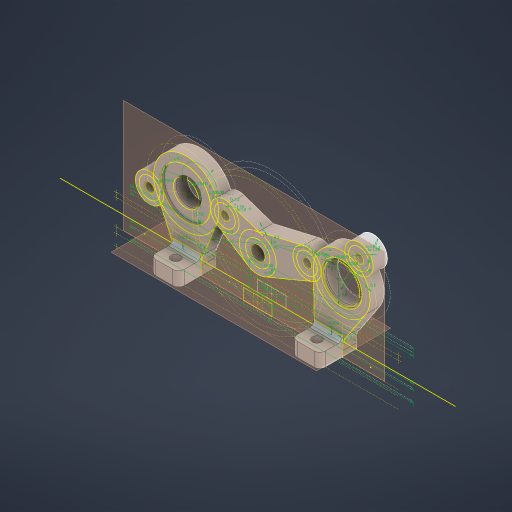
# Autodesk Inventor part: Motormount
Saved by Autodesk Inventor 2023.5 (Build 275446000, 446)
## iProperties
Created: 2024-12-07
Part Number: Motormount
Material: 一般
Document SubType Name: Modeling
Designer: IshiiLabHonda
Density: 1 g/cm^3
Appearance: 既定
Author: IshiiLabHonda
Autodesk Inventor part; units mm, degrees
ref_plane "YZ Plane" through (0, 0, 0) normal (1, 0, 0) x (0, 1, 0)
ref_plane "XZ Plane" through (0, 0, 0) normal (0, 1, 0) x (-1, 0, 0)
ref_plane "XY Plane" through (0, 0, 0) normal (0, 0, 1) x (1, 0, 0)
sketch "blueprint" plane through (0, 0, 0) normal (0, 0, 1) x (1, 0, 0)
  line L0 (0, 0) -> (0, 1) construction
  line L1 (0, 0) -> (1, 0) construction
  circle A0 centre (0, 0) radius 1.25
  circle A1 centre (0, 0) radius 11.5 construction
  line L2 (-25, -11.5) -> (25, -11.5) construction
  line L3 (-25, -9.5) -> (25, -9.5) construction
  line L4 (-25, -8.5) -> (25, -8.5) construction
  line L5 (-25, -4) -> (25, -4) construction
  circle A2 centre (0, 0) radius 10.65 construction
  circle A3 centre (-12.6949, 2.8) radius 2.25
  circle A4 centre (14.8381, 2.8) radius 4.35 construction
  circle A5 centre (14.8381, 2.8) radius 3.5 construction
  line L6 (-25, -3.2) -> (25, -3.2) construction
  circle A6 centre (-12.6949, 2.8) radius 4.25 construction
  circle A7 centre (-19.1553, 0.4486) radius 0.625 construction
  circle A8 centre (-5.8199, 2.8) radius 0.625 construction
  circle A9 centre (-12.6949, 2.8) radius 6.875 construction
  circle A10 centre (-19.1553, 0.4486) radius 1.825
  circle A11 centre (-5.8199, 2.8) radius 1.825
  circle A12 centre (14.8381, 2.8) radius 5
  circle A13 centre (14.8381, 2.8) radius 6.125 construction
  circle A14 centre (17.9006, 8.1044) radius 0.625 construction
  circle A15 centre (8.7131, 2.8) radius 0.625 construction
  circle A16 centre (17.9006, 8.1044) radius 1.825
  circle A17 centre (-19.1553, 0.4486) radius 0.8
  circle A18 centre (-5.8199, 2.8) radius 0.8
  circle A19 centre (17.9006, 8.1044) radius 0.8
  circle A20 centre (-19.1553, 0.4486) radius 2.5
  circle A21 centre (-5.8199, 2.8) radius 2.5
  circle A22 centre (17.9006, 8.1044) radius 2.5
  circle A23 centre (14.8381, 2.8) radius 3.6
  circle A24 centre (0, 0) radius 3.25
  line L7 (-15, -4) -> (-15, -8.5) construction
  line L8 (15, -4) -> (15, -8.5) construction
  line L9 (-10, -8.5) -> (-10, -6)
  line L10 (-15, -8.5) -> (-15, -6)
  line L11 (-15, -6) -> (-10, -6)
  line L12 (-12.5, -6) -> (-12.5, -8.5)
  line L13 (-13.3, -6) -> (-13.3, -8.5)
  line L14 (-11.7, -6) -> (-11.7, -8.5)
  line L15 (10, -8.5) -> (10, -6)
  line L16 (15, -8.5) -> (15, -6)
  line L17 (15, -6) -> (10, -6)
  line L18 (12.5, -6) -> (12.5, -8.5)
  line L19 (13.3, -6) -> (13.3, -8.5)
  line L20 (11.7, -6) -> (11.7, -8.5)
  line L21 (-15, -8.5) -> (-10, -8.5)
  line L22 (10, -8.5) -> (15, -8.5)
  circle A25 centre (8.7131, 2.8) radius 1.825
  line L23 (-12.6949, 2.8) -> (-19.1553, 0.4486) construction
  line L24 (-12.6949, 2.8) -> (-5.8199, 2.8) construction
  line L25 (14.8381, 2.8) -> (8.7131, 2.8) construction
  circle A26 centre (-12.6949, 2.8) radius 5.75
  line L26 (-2.5, -6.5) -> (2.5, -6.5)
  line L27 (2.5, -6.5) -> (2.5, -8.5)
  line L28 (2.5, -8.5) -> (-2.5, -8.5)
  line L29 (-2.5, -8.5) -> (-2.5, -6.5)
  line L30 (-2.5, -6.5) -> (2.5, -8.5) construction
  line L31 (2.5, -6.5) -> (-2.5, -8.5) construction
  line L32 (0, -6.5) -> (0, -8.5) construction
  line L33 (-0.8, -6.5) -> (-0.8, -8.5) construction
  line L34 (0.8, -6.5) -> (0.8, -8.5) construction
  circle A27 centre (8.7131, 2.8) radius 0.8
  circle A28 centre (8.7131, 2.8) radius 2.5
  line L35 (17.9006, 8.1044) -> (14.8381, 2.8) construction
  circle A29 centre (0, 0) radius 2.15
  circle A30 centre (14.8381, 2.8) radius 3 construction
  circle A31 centre (14.8381, 2.8) radius 3.2
  circle A32 centre (-12.6949, 2.8) radius 4.35
  point P0 (18.8457, 5.7899)
  point P1 (15.4237, 7.7656)
  point P2 (0, -8.5)
  point P3 (-6.4807, -9.5)
  point P4 (6.4807, -9.5)
  point P5 (0, -7.5)
  point P6 (-17.0702, -0.9308)
  point P7 (-7.3074, 0.7907)
  point P8 (-7.3074, 4.8093)
  point P9 (-18.4447, 2.8455)
  point P10 (11.284, 2.5721)
  point P11 (11.284, 2.0279)
  point P12 (16.9793, 5.3162)
  point P13 (16.5081, 5.5882)
  dimension "d0" = 1
  dimension "d1" = 1
  dimension "d2" = 2.5
  dimension "d3" = 23
  dimension "d4" = 50
  dimension "d5" = 50
  dimension "d6" = 2
  dimension "d7" = 50
  dimension "d9" = 1
  dimension "d10" = 50
  dimension "d12" = 4.5
  dimension "d13" = 21.3
  dimension "d14" = 4.5
  dimension "d15" = 8.7
  dimension "d17" = 0.1
  dimension "d18" = 0.1
  dimension "d20" = 7
  dimension "d21" = 50
  dimension "d22" = 0.8
  dimension "d23" = 8.5
  dimension "d26" = 1.25
  dimension "d27" = 1.25
  dimension "d28" = 1.2
  dimension "d29" = 1.2
  dimension "d31" = 1.5
  dimension "d32" = 1.25
  dimension "d33" = 1.25
  dimension "d34" = 1.2
  dimension "d37" = 0.5
  dimension "d40" = 1.6
  dimension "d41" = 1.6
  dimension "d43" = 1.6
  dimension "d49" = 2
  dimension "d56" = 30
  dimension "d90" = 2.5
  dimension "d92" = 5
  dimension "d93" = 1.6
  dimension "d104" = 1.2
  dimension "d105" = 5
  dimension "d106" = 1.6
  dimension "d107" = 2.5
  dimension "d129" = 5
  dimension "d130" = 5
  dimension "d132" = 5
  dimension "d155" = 25
  dimension "d158" = 1.5
  dimension "d160" = 0.5
  dimension "d161" = 200
  dimension "d166" = 1.6
  dimension "d167" = 5
  dimension "d168" = 2
  dimension "d178" = 1.6
  dimension "d179" = 5
  dimension "d181" = 6
  dimension "d187" = 1.75
  dimension "d196" = 4.3
  dimension "d218" = 10.6088
  dimension "d219" = 13.5411
  dimension "d220" = 120
  dimension "d221" = 6
  dimension "d237" = 0.1
  dimension "d238" = 6
  dimension "d239" = 0.2
  dimension "d247" = 0.1
  constraints: 70 end point, 33 centre point, 28 coincident, 16 point on line, 10 parallel, 8 midpoint, 7 vertical, 6 point on circle, 5 symmetric about line, 4 perpendicular, 3 horizontal, 1 tangent, 18 other
  measures "d0" distance of L0.start L0.end
  measures "d1" distance of L0.start L1.end
  measures "d2" diameter of A0
  measures "d3" diameter of A1
  measures "d4" distance of L2.start L2.end
  measures "d5" distance of L3.start L3.end
  measures "d6" distance between parallel lines of L2 L3
  measures "d7" distance of point (-25, -8.5) point (25, -8.5)
  measures "d10" distance of L5.start L5.end
  measures "d13" diameter of A2
  measures "d14" diameter of A3
  measures "d15" diameter of A4
  measures "d20" diameter of A5
  measures "d21" distance of L6.start L6.end
  measures "d22" distance between parallel lines of L5 L6
  measures "d23" diameter of A6
  measures "d26" diameter of A8
  measures "d27" diameter of A7
  measures "d28" radial gap between concentric circles of A10 A7
  measures "d29" radial gap between concentric circles of A11 A8
  measures "d31" radial gap between concentric circles of A12 A5
  measures "d32" diameter of A14
  measures "d33" diameter of A15
  measures "d34" radial gap between concentric circles of A14 A16
  measures "d40" diameter of A17
  measures "d41" diameter of A18
  measures "d43" diameter of A19
  measures "d49" radial gap between concentric circles of A24 A0
  measures "d56" distance between parallel lines of L8 L7
  measures "d90" distance of L10.start L10.end
  measures "d92" distance between parallel lines of L9 L10
  measures "d93" distance between parallel lines of L14 L13
  measures "d104" radial gap between concentric circles of A25 A15
  measures "d105" distance between parallel lines of L16 L15
  measures "d106" distance between parallel lines of L19 L20
  measures "d107" distance of L15.start L15.end
  measures "d129" diameter of A20
  measures "d130" diameter of A21
  measures "d132" diameter of A22
  measures "d155" distance between parallel lines of L18 L12
  measures "d158" radial gap between concentric circles of A26 A6
  measures "d166" distance between parallel lines of L33 L34
  measures "d167" distance between parallel lines of L27 L29
  measures "d168" distance between parallel lines of L26 L28
  measures "d178" diameter of A27
  measures "d179" diameter of A28
  measures "d181" distance between parallel lines of L6 L25
  measures "d187" distance edge to line of A6 L6
  measures "d196" diameter of A29
  measures "d218" distance of A14.centre L25.end
  measures "d219" distance of A7.centre A18.centre
  measures "d220" angle of L25 L35
  measures "d221" distance from line of A3.centre L6
  measures "d237" radial gap between concentric circles of A5 A23
  measures "d238" diameter of A30
  measures "d239" radial gap between concentric circles of A30 A31
  measures "d247" radial gap between concentric circles of A6 A32
sketch "スケッチ5" plane through (0, 0, 0) normal (0, 0, 1) x (1, 0, 0)
  circle A0 centre (0, 0) radius 10.65 construction
  circle A1 centre (0, 0) radius 11.5 construction
  line L0 (-25, -3.2) -> (25, -3.2) construction
  line L1 (-25, -4) -> (25, -4) construction
  line L2 (-25, -8.5) -> (25, -8.5) construction
  line L3 (-25, -9.5) -> (25, -9.5) construction
  line L4 (-25, -11.5) -> (25, -11.5) construction
  line L5 (0, 0) -> (1, 0) construction
  circle A2 centre (0, 0) radius 1.25 projected
  line L6 (0, 0) -> (0, 1) construction
  circle A3 centre (-5.8199, 2.8) radius 0.625 construction
  circle A4 centre (-5.8199, 2.8) radius 0.8 projected
  circle A5 centre (-5.8199, 2.8) radius 1.825 construction
  circle A6 centre (-5.8199, 2.8) radius 2.5 projected
  line L7 (-12.6949, 2.8) -> (-5.8199, 2.8) construction
  circle A7 centre (-12.6949, 2.8) radius 2.25 projected
  circle A8 centre (-12.6949, 2.8) radius 4.25 construction
  circle A9 centre (-12.6949, 2.8) radius 5.75 projected
  circle A10 centre (-12.6949, 2.8) radius 6.875 construction
  line L8 (-12.6949, 2.8) -> (-19.1553, 0.4486) construction
  circle A11 centre (-19.1553, 0.4486) radius 2.5 projected
  circle A12 centre (14.8381, 2.8) radius 3.5 construction
  circle A13 centre (14.8381, 2.8) radius 4.35 construction
  circle A14 centre (-19.1553, 0.4486) radius 0.625 construction
  circle A15 centre (-19.1553, 0.4486) radius 0.8 projected
  circle A16 centre (-19.1553, 0.4486) radius 1.825 construction
  circle A17 centre (14.8381, 2.8) radius 5 projected
  circle A18 centre (14.8381, 2.8) radius 6.125 construction
  circle A19 centre (17.9006, 8.1044) radius 0.625 construction
  circle A20 centre (8.7131, 2.8) radius 0.625 construction
  circle A21 centre (17.9006, 8.1044) radius 1.825 construction
  line L9 (14.8381, 2.8) -> (8.7131, 2.8) construction
  circle A22 centre (8.7131, 2.8) radius 0.8 projected
  circle A23 centre (8.7131, 2.8) radius 1.825 construction
  circle A24 centre (8.7131, 2.8) radius 2.5 projected
  circle A25 centre (14.8381, 2.8) radius 3.6 projected
  line L10 (17.9006, 8.1044) -> (14.8381, 2.8) construction
  circle A26 centre (17.9006, 8.1044) radius 2.5 projected
  circle A27 centre (17.9006, 8.1044) radius 0.8 projected
  line L11 (-10, -8.5) -> (-10, -6) projected
  line L12 (-11.7, -6) -> (-11.7, -8.5) projected
  line L13 (-15, -6) -> (-10, -6) projected
  line L14 (-12.5, -6) -> (-12.5, -8.5) projected
  line L15 (-13.3, -6) -> (-13.3, -8.5) projected
  line L16 (-15, -8.5) -> (-10, -8.5) projected
  line L17 (-15, -4) -> (-15, -8.5) construction
  line L18 (-15, -8.5) -> (-15, -6) projected
  line L19 (15, -4) -> (15, -8.5) construction
  line L20 (15, -8.5) -> (15, -6) projected
  line L21 (13.3, -6) -> (13.3, -8.5) projected
  line L22 (15, -6) -> (10, -6) projected
  line L23 (12.5, -6) -> (12.5, -8.5) projected
  line L24 (11.7, -6) -> (11.7, -8.5) projected
  line L25 (10, -8.5) -> (15, -8.5) projected
  line L26 (10, -8.5) -> (10, -6) projected
  circle A28 centre (0, 0) radius 3.25 projected
  line L27 (-2.5, -8.5) -> (-2.5, -6.5) projected
  line L28 (-0.8, -6.5) -> (-0.8, -8.5) construction
  line L29 (0, -6.5) -> (0, -8.5) construction
  line L30 (0.8, -6.5) -> (0.8, -8.5) construction
  line L31 (-2.5, -6.5) -> (2.5, -6.5) projected
  line L32 (-2.5, -6.5) -> (2.5, -8.5) construction
  line L33 (2.5, -6.5) -> (-2.5, -8.5) construction
  line L34 (2.5, -8.5) -> (-2.5, -8.5) projected
  line L35 (2.5, -6.5) -> (2.5, -8.5) projected
  line L36 (-15, -6) -> (-17.9261, 0.4132)
  line L37 (-10, -6) -> (-7.3501, 0.6797)
  line L38 (10, -6) -> (9.839, 2.7076)
  line L39 (15, -6) -> (19.0045, 0.0357)
  line L40 (-7.158, 0.6883) -> (-1.7396, -2.7452)
  line L41 (-5.005, 5.1635) -> (1.0594, 3.0725)
  line L42 (-0.7374, 3.1652) -> (8.1459, 5.2348)
  line L43 (1.2445, -3.0023) -> (9.6705, 0.4906)
  point P0 (0, -7.5)
  point P1 (0, -8.5)
  point P2 (6.4807, -9.5)
  point P3 (-6.4807, -9.5)
  point P4 (10.245, 0.8243)
  point P5 (9.8782, 0.5881)
  point P6 (0.1743, 3.3777)
  point P7 (-18.4447, 2.8455)
  point P8 (-17.0702, -0.9308)
  point P9 (-7.3074, 0.7907)
  point P10 (18.8457, 5.7899)
  point P11 (15.4237, 7.7656)
  point P12 (10.245, 4.7757)
  point P13 (-7.3074, 4.8093)
  point P14 (18.0158, -1.9266)
  point P15 (-17.2201, -1.1342)
  constraints: 16 end point, 12 point on circle, 12 tangent, 5 other
extrude "押し出し33" add sketch "スケッチ5" along normal blind 2.5 contours A6 A9 | A6 L41 L42 A28 L40 | A9 A6 | A6 A9 A11 | L42 A24 L43 A28 L41 | L41 A28 L42 | A28 | A11 A9 | A9 L36 A11 | A24 A17 L38 | L37 L13 L36 A11 A9 | A9 A11 L36 | A24 A17 | A17 A26 A24 | L11 L16 L12 L13 | L13 L15 L16 L18 | L38 A17 A24 | A24 A17 L39 L22 L38 | A26 A17 | A17 A26 | L12 L16 L14 L13 | L13 L14 L16 L15 | L22 L24 L25 L26 | L22 L23 L25 L24 | L20 L25 L21 L22 | L22 L21 L25 L23 | A25 | A27
extrude "押し出し34" cut sketch "blueprint" along normal blind 0.5 contours A10 A26 | A26 A10 | A26 A11 | A11 A26 | A16 A12 | A12 A16 | A25 A12 | A12 A25 | A17 | A19 | A29
fillet "フィレット7" radius 5 3 edges at (15, -6, 1.25) (-15, -6, 1.25) (-10, -6, 1.25)
extrude "押し出し39" add sketch "blueprint" along normal blind 6.5 contours L21 L14 L11 L9 | L21 L12 L11 L14 | L21 L13 L11 L12 | L21 L10 L11 L13 | L15 L17 L20 L22 | L20 L17 L18 L22 | L18 L17 L19 L22 | L19 L17 L16 L22
ref_plane "作業平面8" through (-15, -6, 2.5) normal (0, 1, 0) x (1, 0, 0)
sketch "スケッチ9" plane through (-15, -6, 2.5) normal (0, 1, 0) x (1, 0, 0)
  line L0 (0, 0) -> (5, 0) projected
  line L1 (0, 0) -> (0, -4) projected
  line L2 (5, -4) -> (0, -4) projected
  line L3 (5, 0) -> (5, -4) projected
  line L4 (25, 0) -> (30, 0) projected
  line L5 (25, 0) -> (25, -4) projected
  line L6 (30, -4) -> (25, -4) projected
  line L7 (30, 0) -> (30, -4) projected
  line L8 (0, 2.5) -> (0, 0) projected
  line L9 (5, 2.5) -> (5, -4) projected
  line L10 (0, 0) -> (5, -4) construction
  line L11 (0, 2.5) -> (0, -4) projected
  line L12 (5, 0) -> (5.3524, 0) projected
  line L13 (0, -4) -> (5, 0) construction
  line L14 (30, 2.5) -> (30, -4) projected
  line L15 (25, 0) -> (30, -4) construction
  line L16 (25, 2.5) -> (25, -4) projected
  line L17 (30, 0) -> (30, 2.5) projected
  line L18 (25, -4) -> (30, 0) construction
  circle A0 centre (2.5, -2) radius 0.8
  circle A1 centre (27.5, -2) radius 0.8
  point P0 (15, 2.5)
  dimension "d227" = 1.6
  dimension "d228" = 1.6
  constraints: 8 end point, 2 centre point, 2 midpoint
  measures "d227" diameter of A0
  measures "d228" diameter of A1
extrude "押し出し40" cut sketch "スケッチ9" against normal blind 6.5 contours A0 | A1
fillet "フィレット8" radius 1 4 edges at (-15, -7.25, 6.5) (-10, -7.25, 6.5) (10, -7.25, 6.5) (15, -7.25, 6.5)
fillet "フィレット9" radius 0.8 2 edges at (-12.5, -6, 2.5) (12.5, -6, 2.5)
extrude "押し出し41" cut sketch "スケッチ5" along normal blind 6.5 contours A27
extrude "押し出し42" cut sketch "blueprint" along normal blind 6.5 contours A23 | A31
extrude "押し出し43" add sketch "blueprint" along normal up to surface (2.5 mm away) contours A23
ref_plane "作業平面9" through (0, 0, 2.5) normal (0, 0, 1) x (1, 0, 0)
sketch "スケッチ10" plane through (0, 0, 2.5) normal (0, 0, 1) x (1, 0, 0)
  line L0 (8.1459, 5.2348) -> (0.1743, 3.3777) projected
  line L1 (0.1743, 3.3777) -> (-5.005, 5.1635) projected
  arc A0 (-5.005, 5.1635) -> (-7.3074, 4.8093) centre (-5.8199, 2.8) ccw projected
  line L2 (0.1743, 3.3777) -> (-5.005, 5.1635) projected
  line L3 (-7.158, 0.6883) -> (-1.7396, -2.7452) projected
  line L4 (-7.158, 0.6883) -> (-1.7396, -2.7452) projected
  circle A1 centre (-5.8199, 2.8) radius 0.8 projected
  circle A2 centre (-5.8199, 2.8) radius 0.8 projected
  circle A3 centre (-5.8199, 2.8) radius 1.825 projected
  circle A4 centre (-5.8199, 2.8) radius 1.825 projected
  arc A5 (-5.005, 5.1635) -> (-7.3074, 4.8093) centre (-5.8199, 2.8) ccw projected
  arc A6 (-7.3074, 0.7907) -> (-7.158, 0.6883) centre (-5.8199, 2.8) ccw projected
  arc A7 (-7.3501, 0.6797) -> (-7.3074, 0.7907) centre (-12.6949, 2.8) ccw projected
  arc A8 (-7.3074, 0.7907) -> (-7.158, 0.6883) centre (-5.8199, 2.8) ccw projected
  arc A9 (-7.3501, 0.6797) -> (-7.3074, 0.7907) centre (-12.6949, 2.8) ccw projected
  arc A10 (-1.7396, -2.7452) -> (1.2445, -3.0023) centre (0, 0) ccw projected
  circle A11 centre (0, 0) radius 1.25 projected
  circle A12 centre (0, 0) radius 1.25 projected
  circle A13 centre (0, 0) radius 2.15 projected
  circle A14 centre (0, 0) radius 2.15 projected
  line L5 (0.1743, 3.3777) -> (-5.005, 5.1635) projected
  arc A15 (-1.7396, -2.7452) -> (1.2445, -3.0023) centre (0, 0) ccw projected
  line L6 (8.1459, 5.2348) -> (0.1743, 3.3777) projected
  arc A16 (-1.7396, -2.7452) -> (1.2445, -3.0023) centre (0, 0) ccw projected
  arc A17 (-1.7396, -2.7452) -> (1.2445, -3.0023) centre (0, 0) ccw projected
  line L7 (1.2445, -3.0023) -> (9.6705, 0.4906) projected
  line L8 (8.1459, 5.2348) -> (0.1743, 3.3777) projected
  line L9 (0.1743, 3.3777) -> (-5.005, 5.1635) projected
  line L10 (8.1459, 5.2348) -> (0.1743, 3.3777) projected
  circle A18 centre (8.7131, 2.8) radius 0.8 projected
  circle A19 centre (8.7131, 2.8) radius 0.8 projected
  line L11 (1.2445, -3.0023) -> (9.6705, 0.4906) projected
  line L12 (-15, -8.5) -> (-10, -8.5) projected
  line L13 (-10, -8.5) -> (-10, -6.9556) projected
  line L14 (-10, -6) -> (-10, -5.2) projected
  arc A20 (-15, -7.0868) -> (-15.4511, -5.0113) centre (-20, -7.0868) ccw projected
  arc A21 (-15, -7.0868) -> (-15.4511, -5.0113) centre (-20, -7.0868) ccw projected
  line L15 (-15, -7.0868) -> (-15, -5.2) projected
  line L16 (-10, -8.5) -> (-10, -6) projected
  line L17 (-15, -5.2) -> (-15, -6) projected
  line L18 (-15, -6) -> (-10, -6) projected
  line L19 (-11, -6) -> (-11, -8.5) projected
  line L20 (-10, -8.5) -> (-11, -8.5) projected
  line L21 (-11, -6) -> (-14, -6) projected
  line L22 (-14, -8.5) -> (-11, -8.5) projected
  line L23 (-15, -6) -> (-15, -8.5) projected
  line L24 (-14, -8.5) -> (-14, -6) projected
  line L25 (-15, -6) -> (-14, -6) projected
  line L26 (-15, -7.0868) -> (-15, -8.5) projected
  arc A22 (9.6705, 0.4906) -> (9.8782, 0.5881) centre (8.7131, 2.8) ccw projected
  arc A23 (19.0045, 0.0357) -> (18.8457, 5.7899) centre (14.8381, 2.8) ccw projected
  arc A24 (18.8457, 5.7899) -> (15.4237, 7.7656) centre (17.9006, 8.1044) ccw projected
  arc A25 (15.4237, 7.7656) -> (10.245, 4.7757) centre (14.8381, 2.8) ccw projected
  arc A26 (10.245, 4.7757) -> (8.1459, 5.2348) centre (8.7131, 2.8) ccw projected
  circle A27 centre (17.9006, 8.1044) radius 1.825 projected
  circle A28 centre (17.9006, 8.1044) radius 1.825 projected
  circle A29 centre (14.8381, 2.8) radius 3.2 projected
  circle A30 centre (14.8381, 2.8) radius 3.2 projected
  arc A31 (19.0045, 0.0357) -> (18.8457, 5.7899) centre (14.8381, 2.8) ccw projected
  arc A32 (10.245, 4.7757) -> (8.1459, 5.2348) centre (8.7131, 2.8) ccw projected
  arc A33 (15.4237, 7.7656) -> (10.245, 4.7757) centre (14.8381, 2.8) ccw projected
  circle A34 centre (17.9006, 8.1044) radius 0.8 projected
  arc A35 (18.8457, 5.7899) -> (15.4237, 7.7656) centre (17.9006, 8.1044) ccw projected
  circle A36 centre (17.9006, 8.1044) radius 0.8 projected
  line L27 (-10, -5.2) -> (-10, -6.9556) projected
  arc A37 (-9.6476, -5.1118) -> (-10, -6.9556) centre (-5, -6.9556) ccw projected
  arc A38 (-9.6476, -5.1118) -> (-10, -6.9556) centre (-5, -6.9556) ccw projected
  line L28 (-14, -8.5) -> (-15, -8.5) projected
  line L29 (-11.7, -8.5) -> (-13.3, -8.5) projected
  line L30 (-13.3, -6) -> (-11.7, -6) projected
  line L31 (9.8782, 0.5881) -> (10, -6) projected
  line L32 (10, -8.5) -> (15, -8.5) projected
  line L33 (15, -8.5) -> (15, -7.5078) projected
  line L34 (15.8336, -4.7436) -> (19.0045, 0.0357) projected
  arc A39 (15.8336, -4.7436) -> (15, -7.5078) centre (20, -7.5078) ccw projected
  line L35 (15.8336, -4.7436) -> (19.0045, 0.0357) projected
  arc A40 (9.6705, 0.4906) -> (9.8782, 0.5881) centre (8.7131, 2.8) ccw projected
  line L36 (15, -6) -> (15, -5.2) projected
  line L37 (9.8782, 0.5881) -> (9.9852, -5.2) projected
  arc A41 (15.8336, -4.7436) -> (15, -7.5078) centre (20, -7.5078) ccw projected
  line L38 (15, -5.2) -> (15, -7.5078) projected
  line L39 (15, -5.2) -> (9.9852, -5.2) projected
  line L40 (11.7, -6) -> (13.3, -6) projected
  line L41 (10, -6) -> (15, -6) projected
  line L42 (9.9852, -5.2) -> (10, -6) projected
  line L43 (15, -8.5) -> (15, -6) projected
  line L44 (13.3, -8.5) -> (11.7, -8.5) projected
  line L45 (10, -6) -> (10, -8.5) projected
  line L46 (10, -6) -> (10, -8.5) projected
  arc A42 (-7.3074, 4.8093) -> (-18.4447, 2.8455) centre (-12.6949, 2.8) ccw projected
  arc A43 (-18.4447, 2.8455) -> (-17.2201, -1.1342) centre (-19.1553, 0.4486) ccw projected
  line L47 (-17.2201, -1.1342) -> (-15.4511, -5.0113) projected
  circle A44 centre (-12.6949, 2.8) radius 2.25 projected
  circle A45 centre (-19.1553, 0.4486) radius 0.8 projected
  circle A46 centre (-19.1553, 0.4486) radius 1.825 projected
  circle A47 centre (-19.1553, 0.4486) radius 1.825 projected
  circle A48 centre (8.7131, 2.8) radius 1.825 projected
  circle A49 centre (8.7131, 2.8) radius 1.825 projected
  line L48 (-9.6476, -5.1118) -> (-7.3501, 0.6797) projected
  circle A50 centre (-19.1553, 0.4486) radius 0.8 projected
  circle A51 centre (-12.6949, 2.8) radius 2.25 projected
  line L49 (-9.6476, -5.1118) -> (-7.3501, 0.6797) projected
  arc A52 (-7.3074, 4.8093) -> (-18.4447, 2.8455) centre (-12.6949, 2.8) ccw projected
  line L50 (-17.2201, -1.1342) -> (-15.4511, -5.0113) projected
  arc A53 (-18.4447, 2.8455) -> (-17.2201, -1.1342) centre (-19.1553, 0.4486) ccw projected
  line L51 (-10, -5.2) -> (-15, -5.2) projected
  line L52 (-11, -6) -> (-10, -6) projected
  line L53 (11, -8.5) -> (10, -8.5) projected
  line L54 (11, -8.5) -> (14, -8.5) projected
  line L55 (11, -8.5) -> (11, -6) projected
  line L56 (15, -8.5) -> (14, -8.5) projected
  line L57 (14, -6) -> (14, -8.5) projected
  line L58 (14, -6) -> (15, -6) projected
  line L59 (14, -6) -> (11, -6) projected
  line L60 (10, -6) -> (11, -6) projected
  line L61 (-35, -6) -> (35, -6) projected
  line L62 (-25, -3.2) -> (25, -3.2) construction
  line L63 (-25, -4) -> (25, -4) construction
  line L64 (-25, -8.5) -> (25, -8.5) construction
  line L65 (-25, -9.5) -> (25, -9.5) construction
  line L66 (-25, -11.5) -> (25, -11.5) construction
  circle A54 centre (0, 0) radius 10.65 construction
  circle A55 centre (0, 0) radius 11.5 construction
  circle A56 centre (0, 0) radius 1.25 projected
  circle A57 centre (0, 0) radius 3.25 projected
  line L67 (-2.5, -8.5) -> (-2.5, -6.5) projected
  line L68 (-0.8, -6.5) -> (-0.8, -8.5) construction
  circle A58 centre (0, 0) radius 2.15 projected
  line L69 (0, -6.5) -> (0, -8.5) construction
  line L70 (0.8, -6.5) -> (0.8, -8.5) construction
  line L71 (-2.5, -6.5) -> (2.5, -6.5) projected
  line L72 (2.5, -8.5) -> (-2.5, -8.5) projected
  line L73 (2.5, -6.5) -> (-2.5, -8.5) construction
  line L74 (-2.5, -6.5) -> (2.5, -8.5) construction
  circle A59 centre (-5.8199, 2.8) radius 0.625 construction
  circle A60 centre (-5.8199, 2.8) radius 0.8 projected
  circle A61 centre (-5.8199, 2.8) radius 1.825 projected
  circle A62 centre (-5.8199, 2.8) radius 2.5 projected
  line L75 (-15, -4) -> (-15, -8.5) construction
  line L76 (-15, -8.5) -> (-15, -6) projected
  line L77 (-13.3, -6) -> (-13.3, -8.5) projected
  line L78 (-12.5, -6) -> (-12.5, -8.5) projected
  line L79 (-15, -6) -> (-10, -6) projected
  line L80 (-11.7, -6) -> (-11.7, -8.5) projected
  line L81 (-15, -8.5) -> (-10, -8.5) projected
  line L82 (-10, -8.5) -> (-10, -6) projected
  circle A63 centre (-12.6949, 2.8) radius 2.25 projected
  circle A64 centre (-12.6949, 2.8) radius 4.25 construction
  line L83 (-12.6949, 2.8) -> (-5.8199, 2.8) construction
  circle A65 centre (-12.6949, 2.8) radius 5.75 projected
  circle A66 centre (-12.6949, 2.8) radius 6.875 construction
  line L84 (-12.6949, 2.8) -> (-19.1553, 0.4486) construction
  circle A67 centre (-19.1553, 0.4486) radius 0.625 construction
  circle A68 centre (-19.1553, 0.4486) radius 1.825 projected
  circle A69 centre (-19.1553, 0.4486) radius 2.5 projected
  circle A70 centre (-19.1553, 0.4486) radius 0.8 projected
  line L85 (2.5, -6.5) -> (2.5, -8.5) projected
  line L86 (15, -6) -> (10, -6) projected
  line L87 (10, -8.5) -> (10, -6) projected
  line L88 (10, -8.5) -> (15, -8.5) projected
  line L89 (15, -4) -> (15, -8.5) construction
  line L90 (15, -8.5) -> (15, -6) projected
  line L91 (11.7, -6) -> (11.7, -8.5) projected
  line L92 (12.5, -6) -> (12.5, -8.5) projected
  line L93 (13.3, -6) -> (13.3, -8.5) projected
  circle A71 centre (14.8381, 2.8) radius 5 projected
  circle A72 centre (14.8381, 2.8) radius 6.125 construction
  circle A73 centre (17.9006, 8.1044) radius 0.625 construction
  circle A74 centre (8.7131, 2.8) radius 0.625 construction
  circle A75 centre (17.9006, 8.1044) radius 1.825 projected
  circle A76 centre (17.9006, 8.1044) radius 0.8 projected
  circle A77 centre (17.9006, 8.1044) radius 2.5 projected
  line L94 (14.8381, 2.8) -> (8.7131, 2.8) construction
  circle A78 centre (8.7131, 2.8) radius 1.825 projected
  circle A79 centre (8.7131, 2.8) radius 2.5 projected
  circle A80 centre (14.8381, 2.8) radius 3 construction
  circle A81 centre (14.8381, 2.8) radius 3.2 projected
  circle A82 centre (14.8381, 2.8) radius 3.6 projected
  line L95 (17.9006, 8.1044) -> (14.8381, 2.8) construction
  circle A83 centre (8.7131, 2.8) radius 0.8 projected
  line L96 (0, 0) -> (0, 1) construction
  line L97 (0, 0) -> (1, 0) construction
  circle A84 centre (14.8381, 2.8) radius 3.5 construction
  circle A85 centre (14.8381, 2.8) radius 4.35 construction
  line L98 (12.5, -6) -> (12.5, -8.5) projected
  line L99 (11.7, -6) -> (11.7, -8.5) projected
  line L100 (13.3, -6) -> (13.3, -8.5) projected
  line L101 (10, -8.5) -> (10, -6) projected
  line L102 (10, -8.5) -> (15, -8.5) projected
  line L103 (15, -4) -> (15, -8.5) construction
  line L104 (15, -6) -> (10, -6) projected
  line L105 (15, -6) -> (19.0045, 0.0357) projected
  line L106 (10, -6) -> (9.839, 2.7076) projected
  line L107 (14.8381, 2.8) -> (8.7131, 2.8) construction
  line L108 (1.2445, -3.0023) -> (9.6705, 0.4906) projected
  line L109 (-0.7374, 3.1652) -> (8.1459, 5.2348) projected
  circle A86 centre (0, 0) radius 10.65 construction
  circle A87 centre (0, 0) radius 11.5 construction
  line L110 (-25, -11.5) -> (25, -11.5) construction
  line L111 (-25, -9.5) -> (25, -9.5) construction
  line L112 (-25, -8.5) -> (25, -8.5) construction
  line L113 (-25, -4) -> (25, -4) construction
  line L114 (-25, -3.2) -> (25, -3.2) construction
  circle A88 centre (8.7131, 2.8) radius 0.625 construction
  circle A89 centre (8.7131, 2.8) radius 0.8 projected
  circle A90 centre (8.7131, 2.8) radius 1.825 construction
  circle A91 centre (8.7131, 2.8) radius 2.5 projected
  line L115 (-15, -6) -> (-17.9261, 0.4132) projected
  line L116 (-10, -6) -> (-7.3501, 0.6797) projected
  line L117 (-12.6949, 2.8) -> (-5.8199, 2.8) construction
  circle A92 centre (-19.1553, 0.4486) radius 0.625 construction
  circle A93 centre (-19.1553, 0.4486) radius 0.8 projected
  circle A94 centre (-19.1553, 0.4486) radius 1.825 construction
  circle A95 centre (-19.1553, 0.4486) radius 2.5 projected
  line L118 (-12.6949, 2.8) -> (-19.1553, 0.4486) construction
  circle A96 centre (-12.6949, 2.8) radius 6.875 construction
  circle A97 centre (-12.6949, 2.8) radius 5.75 projected
  circle A98 centre (-12.6949, 2.8) radius 4.25 construction
  circle A99 centre (-12.6949, 2.8) radius 2.25 projected
  circle A100 centre (14.8381, 2.8) radius 3.5 construction
  circle A101 centre (14.8381, 2.8) radius 4.35 construction
  circle A102 centre (14.8381, 2.8) radius 5 projected
  circle A103 centre (14.8381, 2.8) radius 6.125 construction
  circle A104 centre (17.9006, 8.1044) radius 0.625 construction
  circle A105 centre (17.9006, 8.1044) radius 1.825 construction
  circle A106 centre (14.8381, 2.8) radius 3.6 projected
  line L119 (17.9006, 8.1044) -> (14.8381, 2.8) construction
  circle A107 centre (17.9006, 8.1044) radius 0.8 projected
  circle A108 centre (17.9006, 8.1044) radius 2.5 projected
  line L120 (-15, -6) -> (-10, -6) projected
  line L121 (-15, -4) -> (-15, -8.5) construction
  line L122 (-15, -8.5) -> (-10, -8.5) projected
  line L123 (-15, -8.5) -> (-15, -6) projected
  line L124 (-13.3, -6) -> (-13.3, -8.5) projected
  line L125 (-12.5, -6) -> (-12.5, -8.5) projected
  line L126 (-11.7, -6) -> (-11.7, -8.5) projected
  line L127 (-10, -8.5) -> (-10, -6) projected
  line L128 (0, 0) -> (1, 0) construction
  circle A109 centre (0, 0) radius 1.25 projected
  line L129 (0, 0) -> (0, 1) construction
  circle A110 centre (-5.8199, 2.8) radius 0.625 construction
  circle A111 centre (-5.8199, 2.8) radius 0.8 projected
  circle A112 centre (-5.8199, 2.8) radius 1.825 construction
  circle A113 centre (-5.8199, 2.8) radius 2.5 projected
  line L130 (-7.158, 0.6883) -> (-1.7396, -2.7452) projected
  line L131 (-2.5, -8.5) -> (-2.5, -6.5) projected
  line L132 (-0.8, -6.5) -> (-0.8, -8.5) construction
  line L133 (0, -6.5) -> (0, -8.5) construction
  line L134 (0.8, -6.5) -> (0.8, -8.5) construction
  line L135 (-5.005, 5.1635) -> (1.0594, 3.0725) projected
  circle A114 centre (0, 0) radius 3.25 projected
  line L136 (2.5, -6.5) -> (2.5, -8.5) projected
  line L137 (-2.5, -6.5) -> (2.5, -8.5) construction
  line L138 (2.5, -6.5) -> (-2.5, -8.5) construction
  line L139 (2.5, -8.5) -> (-2.5, -8.5) projected
  line L140 (-2.5, -6.5) -> (2.5, -6.5) projected
  line L141 (15, -8.5) -> (15, -6) projected
  circle A115 centre (-12.6949, 2.8) radius 4.35 projected
  point P0 (0, -8.5)
  point P1 (0, -7.5)
  point P2 (6.4807, -9.5)
  point P3 (-6.4807, -9.5)
  point P4 (-6.4807, -9.5)
  point P5 (6.4807, -9.5)
  point P6 (0, -8.5)
  point P7 (0, -7.5)
  constraints: 43 other
extrude "押し出し45" cut sketch "スケッチ10" against normal blind 0.5 contours A82
extrude "押し出し46" cut sketch "スケッチ10" against normal blind 0.5 contours A115
equation "\"d5\" = d4"
equation "\"d7\" = d4"
equation "\"d10\" = d4"
